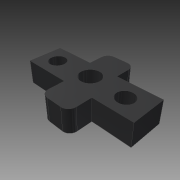
# Autodesk Inventor part: x_motor_lower_nut_stop
Saved by Autodesk Inventor 2014 (Build 180170000, 170)
## iProperties
Created: 2013-12-01
Part Number: x_motor_lower_nut_stop
Material: Generic
Document SubType Name: Modeling
Designer: buben
Density: 1 g/cm^3
Appearance: Anodized - Dark Gray
Author: buben
Subject: Laser Cutted
Autodesk Inventor part; units mm, degrees
ref_plane "YZ Plane" through (0, 0, 0) normal (1, 0, 0) x (0, 1, 0)
ref_plane "XZ Plane" through (0, 0, 0) normal (0, 1, 0) x (-1, 0, 0)
ref_plane "XY Plane" through (0, 0, 0) normal (0, 0, 1) x (1, 0, 0)
sketch "Sketch1" plane through (0, 0, 0) normal (0, 0, 1) x (1, 0, 0)
  line L0 (0, 0) -> (30, 0)
  line L1 (30, 0) -> (30, 9)
  line L2 (30, 9) -> (0, 9)
  line L3 (0, 9) -> (0, 0)
  circle A0 centre (-5.5, 5.099) radius 7.5 construction
  circle A1 centre (-5.5, 5.099) radius 4 construction
  circle A2 centre (14.5, 5.099) radius 2.75
  circle A3 centre (24.5, 4.5) radius 2.25
  circle A4 centre (4.5, 4.5) radius 2.25
  point P0 (-11, 0)
  point P1 (30, 4.5)
  dimension "d0" = 9
  dimension "d1" = 30
  dimension "d2" = 15
  dimension "d3" = 8
  dimension "d4" = 11
  dimension "d5" = 5.5
  dimension "d6" = 4.5
  dimension "d7" = 4.5
  dimension "d8" = 5.5
  dimension "d9" = 10
  dimension "d10" = 10
  constraints: 8 end point, 5 centre point, 4 horizontal alignment, 2 parallel, 2 point on circle, 1 coincident, 1 horizontal, 1 midpoint, 1 perpendicular
  measures "d0" distance of L2.end L0.start
  measures "d1" distance of L0.start L0.end
  measures "d2" diameter of A0
  measures "d3" diameter of A1
  measures "d4" distance of L0.start A0.start
  measures "d5" diameter of A2
  measures "d6" diameter of A3
  measures "d7" diameter of A4
  measures "d8" distance from line of L1 A3.centre
  measures "d9" horizontal distance of A2.centre A3.centre
  measures "d10" horizontal distance of A4.centre A2.centre
extrude "Extrusion1" add sketch "Sketch1" along normal blind 6
sketch "Sketch2" plane through (0, 0, 6) normal (0, 0, 1) x (1, 0, 0)
  line L0 (0, 0) -> (30, 0) projected
  line L1 (30, 0) -> (30, 9) projected
  line L2 (30, 9) -> (0, 9) projected
  line L3 (12, 0) -> (20, 0)
  line L4 (20, 0) -> (20, -4)
  line L5 (18, -6) -> (14, -6)
  line L6 (12, -4) -> (12, 0)
  arc A0 (12, -4) -> (14, -6) centre (14, -4) ccw
  arc A1 (18, -6) -> (20, -4) centre (18, -4) ccw
  line L7 (10.5, 9) -> (18.5, 9)
  line L8 (18.5, 9) -> (18.5, 13)
  line L9 (16.5, 15) -> (12.5, 15)
  line L10 (10.5, 13) -> (10.5, 9)
  arc A2 (12.5, 15) -> (10.5, 13) centre (12.5, 13) ccw
  arc A3 (18.5, 13) -> (16.5, 15) centre (16.5, 13) ccw
  dimension "d13" = 2
  dimension "d14" = 8
  dimension "d15" = 6
  dimension "d16" = 10
  dimension "d17" = 2
  dimension "d18" = 8
  dimension "d19" = 6
  dimension "d20" = 11.5
  constraints: 16 end point, 8 point on circle, 8 tangent, 4 centre point, 4 parallel, 2 equal radius, 2 horizontal, 2 perpendicular, 2 point on line
  measures "d13" radius of A0
  measures "d14" distance between parallel lines of L4 L6
  measures "d15" distance between parallel lines of L0 L5
  measures "d16" distance between parallel lines of L1 L4
  measures "d17" radius of A2
  measures "d18" distance between parallel lines of L8 L10
  measures "d19" distance between parallel lines of L2 L9
  measures "d20" distance between parallel lines of L1 L8
extrude "Extrusion2" add sketch "Sketch2" against normal blind 6
body "Solid1"
